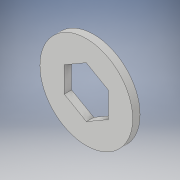
# Autodesk Inventor part: Spacer 1 16 in
Saved by Autodesk Inventor 2018 (Build 220112000, 112)
## iProperties
Created: 2019-01-14
Part Number: Spacer 1 16 in
Material: Generic
Document SubType Name: Modeling
Designer: Gabriel
Density: 1 g/cm^3
Appearance: Default
Author: Gabriel
Autodesk Inventor part; units mm, degrees
ref_plane "YZ Plane" through (0, 0, 0) normal (1, 0, 0) x (0, 1, 0)
ref_plane "XZ Plane" through (0, 0, 0) normal (0, 1, 0) x (-1, 0, 0)
ref_plane "XY Plane" through (0, 0, 0) normal (0, 0, 1) x (1, 0, 0)
sketch "Sketch1" plane through (0, 0, 0) normal (0, 0, 1) x (1, 0, 0)
  circle A0 centre (0, 0) radius 9.9949
  line L0 (0, 0) -> (-4.7625, 0)
  line L1 (-4.7625, 2.7354) -> (-0.0123, 5.4921)
  line L2 (-0.0123, 5.4921) -> (4.7502, 2.7568)
  line L3 (4.7502, 2.7568) -> (4.7625, -2.7354)
  line L4 (4.7625, -2.7354) -> (0.0123, -5.4921)
  line L5 (0.0123, -5.4921) -> (-4.7502, -2.7568)
  line L6 (-4.7502, -2.7568) -> (-4.7625, 2.7354)
  dimension "d1" = 19.9898
  dimension "d4" = 4.7625
  constraints: 14 end point, 1 centre point, 1 coincident, 1 horizontal, 13 other
  measures "d1" diameter of A0
  measures "d4" distance of L0.start L0.end
extrude "Extrusion2" add sketch "Sketch1" along normal blind 1.5875
body "Solid2"
